Autodesk Inventor part; units mm, degrees
(part 2 of 4)
  line L221 (-47.1334, -28.1027) -> (-48.7956, -28.1027)
  spline S277 degree 2 poles (-48.7956, -28.1027) (-48.7956, -28.5202) (-48.3755, -28.9637) (-48.0021, -28.9637) knots 0 0 0 1 2 2 2
  spline S278 degree 2 poles (-48.0021, -28.9637) (-47.8699, -28.9637) (-47.6131, -28.904) (-47.5094, -28.8574) knots 0 0 0 1 2 2 2
  spline S279 degree 2 poles (-47.5094, -28.8574) (-47.4005, -28.8055) (-47.2501, -28.7147) (-47.2008, -28.6732) knots 0 0 0 1 2 2 2
  line L222 (-47.2008, -28.6732) -> (-47.1775, -28.6732)
  line L223 (-47.1775, -28.6732) -> (-47.1775, -29.1141)
  spline S280 degree 2 poles (-47.1775, -29.1141) (-47.2475, -29.1426) (-47.4601, -29.2256) (-47.5431, -29.2489) knots 0 0 0 1 2 2 2
  spline S281 degree 2 poles (-47.5431, -29.2489) (-47.6598, -29.2826) (-47.8517, -29.3164) (-47.9969, -29.3164) knots 0 0 0 1 2 2 2
  spline S282 degree 2 poles (-47.5276, -27.7941) (-47.5327, -27.6308) (-47.6002, -27.3922) (-47.665, -27.3118) knots 0 0 0 1 2 2 2
  spline S283 degree 2 poles (-47.665, -27.3118) (-47.735, -27.2211) (-47.9554, -27.1251) (-48.1188, -27.1251) knots 0 0 0 1 2 2 2
  spline S284 degree 2 poles (-48.1188, -27.1251) (-48.2796, -27.1251) (-48.5052, -27.2211) (-48.5985, -27.3144) knots 0 0 0 1 2 2 2
  spline S285 degree 2 poles (-48.5985, -27.3144) (-48.6893, -27.4104) (-48.7827, -27.6412) (-48.7956, -27.7941) knots 0 0 0 1 2 2 2
  line L224 (-48.7956, -27.7941) -> (-47.5276, -27.7941)
  line L225 (-45.4504, -27.2937) -> (-45.4712, -27.2937)
  spline S286 degree 2 poles (-45.4712, -27.2937) (-45.5178, -27.2807) (-45.619, -27.2755) (-45.689, -27.2755) knots 0 0 0 1 2 2 2
  spline S287 degree 2 poles (-45.689, -27.2755) (-45.8524, -27.2755) (-46.1739, -27.4181) (-46.3191, -27.5582) knots 0 0 0 1 2 2 2
  line L226 (-46.3191, -27.5582) -> (-46.3191, -29.2619)
  line L227 (-46.3191, -29.2619) -> (-46.7237, -29.2619)
  line L228 (-46.7237, -29.2619) -> (-46.7237, -26.8606)
  line L229 (-46.7237, -26.8606) -> (-46.3191, -26.8606)
  line L230 (-46.3191, -26.8606) -> (-46.3191, -27.2185)
  spline S288 degree 2 poles (-46.3191, -27.2185) (-46.0987, -27.0214) (-45.7694, -26.8606) (-45.6138, -26.8606) knots 0 0 0 1 2 2 2
  spline S289 degree 2 poles (-45.6138, -26.8606) (-45.5515, -26.8606) (-45.4893, -26.8658) (-45.4504, -26.8736) knots 0 0 0 1 2 2 2
  line L231 (-45.4504, -26.8736) -> (-45.4504, -27.2937)
  spline S290 degree 2 poles (-44.4105, -29.3086) (-44.7399, -29.3086) (-45.1107, -28.9326) (-45.1107, -28.5254) knots 0 0 0 1 2 2 2
  line L232 (-45.1107, -28.5254) -> (-45.1107, -27.1951)
  line L233 (-45.1107, -27.1951) -> (-45.383, -27.1951)
  line L234 (-45.383, -27.1951) -> (-45.383, -26.8606)
  line L235 (-45.383, -26.8606) -> (-45.1107, -26.8606)
  line L236 (-45.1107, -26.8606) -> (-45.1107, -26.1708)
  line L237 (-45.1107, -26.1708) -> (-44.7062, -26.1708)
  line L238 (-44.7062, -26.1708) -> (-44.7062, -26.8606)
  line L239 (-44.7062, -26.8606) -> (-43.9619, -26.8606)
  line L240 (-43.9619, -26.8606) -> (-43.9619, -27.1951)
  line L241 (-43.9619, -27.1951) -> (-44.7062, -27.1951)
  line L242 (-44.7062, -27.1951) -> (-44.7062, -28.3387)
  spline S291 degree 2 poles (-44.7062, -28.3387) (-44.7062, -28.5202) (-44.6932, -28.7199) (-44.6491, -28.8055) knots 0 0 0 1 2 2 2
  spline S292 degree 2 poles (-44.6491, -28.8055) (-44.6128, -28.8807) (-44.4494, -28.9559) (-44.3094, -28.9559) knots 0 0 0 1 2 2 2
  spline S293 degree 2 poles (-44.3094, -28.9559) (-44.2109, -28.9559) (-44.0267, -28.8963) (-43.9853, -28.8781) knots 0 0 0 1 2 2 2
  line L243 (-43.9853, -28.8781) -> (-43.9619, -28.8781)
  line L244 (-43.9619, -28.8781) -> (-43.9619, -29.2412)
  spline S294 degree 2 poles (-43.9619, -29.2412) (-44.076, -29.2723) (-44.3094, -29.3086) (-44.4105, -29.3086) knots 0 0 0 1 2 2 2
  spline S295 degree 2 poles (-70.97, -33.6982) (-70.97, -34.1183) (-71.4835, -34.5747) (-71.9165, -34.5747) knots 0 0 0 1 2 2 2
  spline S296 degree 2 poles (-71.9165, -34.5747) (-72.0203, -34.5747) (-72.3652, -34.5384) (-72.4818, -34.5125) knots 0 0 0 1 2 2 2
  line L245 (-72.4818, -34.5125) -> (-72.4818, -34.1027)
  line L246 (-72.4818, -34.1027) -> (-72.4585, -34.1027)
  spline S297 degree 2 poles (-72.4585, -34.1027) (-72.3703, -34.1339) (-72.1084, -34.2065) (-71.9736, -34.2065) knots 0 0 0 1 2 2 2
  spline S298 degree 2 poles (-71.9736, -34.2065) (-71.7765, -34.2065) (-71.5405, -34.1157) (-71.4861, -34.0327) knots 0 0 0 1 2 2 2
  spline S299 degree 2 poles (-71.4861, -34.0327) (-71.4264, -33.9471) (-71.3953, -33.6982) (-71.3953, -33.5348) knots 0 0 0 1 2 2 2
  line L247 (-71.3953, -33.5348) -> (-71.3953, -31.6703)
  line L248 (-71.3953, -31.6703) -> (-72.0721, -31.6703)
  line L249 (-72.0721, -31.6703) -> (-72.0721, -31.3306)
  line L250 (-72.0721, -31.3306) -> (-70.97, -31.3306)
  line L251 (-70.97, -31.3306) -> (-70.97, -33.6982)
  spline S300 degree 2 poles (-68.4002, -33.33) (-68.4002, -33.9368) (-68.9836, -34.598) (-69.4712, -34.598) knots 0 0 0 1 2 2 2
  spline S301 degree 2 poles (-69.4712, -34.598) (-69.9716, -34.598) (-70.5447, -33.916) (-70.5447, -33.33) knots 0 0 0 1 2 2 2
  spline S302 degree 2 poles (-70.5447, -33.33) (-70.5447, -32.7283) (-69.9535, -32.0619) (-69.4712, -32.0619) knots 0 0 0 1 2 2 2
  spline S303 degree 2 poles (-69.4712, -32.0619) (-68.9836, -32.0619) (-68.4002, -32.7257) (-68.4002, -33.33) knots 0 0 0 1 2 2 2
  spline S304 degree 2 poles (-68.8177, -33.33) (-68.8177, -32.8632) (-69.1574, -32.4094) (-69.4712, -32.4094) knots 0 0 0 1 2 2 2
  spline S305 degree 2 poles (-69.4712, -32.4094) (-69.7849, -32.4094) (-70.1272, -32.8632) (-70.1272, -33.33) knots 0 0 0 1 2 2 2
  spline S306 degree 2 poles (-70.1272, -33.33) (-70.1272, -33.7838) (-69.7849, -34.2505) (-69.4712, -34.2505) knots 0 0 0 1 2 2 2
  spline S307 degree 2 poles (-69.4712, -34.2505) (-69.16, -34.2505) (-68.8177, -33.7916) (-68.8177, -33.33) knots 0 0 0 1 2 2 2
  spline S308 degree 2 poles (-66.9428, -34.5851) (-67.5185, -34.5851) (-68.1512, -33.9394) (-68.1512, -33.3429) knots 0 0 0 1 2 2 2
  spline S309 degree 2 poles (-68.1512, -33.3429) (-68.1512, -32.7569) (-67.5366, -32.0619) (-67.0413, -32.0619) knots 0 0 0 1 2 2 2
  spline S310 degree 2 poles (-67.0413, -32.0619) (-66.8183, -32.0619) (-66.4734, -32.1916) (-66.3464, -32.329) knots 0 0 0 1 2 2 2
  spline S311 degree 2 poles (-66.3464, -32.329) (-66.2167, -32.4664) (-66.0793, -32.8632) (-66.0793, -33.151) knots 0 0 0 1 2 2 2
  line L252 (-66.0793, -33.151) -> (-66.0793, -33.3715)
  line L253 (-66.0793, -33.3715) -> (-67.7415, -33.3715)
  spline S312 degree 2 poles (-67.7415, -33.3715) (-67.7415, -33.789) (-67.3214, -34.2324) (-66.948, -34.2324) knots 0 0 0 1 2 2 2
  spline S313 degree 2 poles (-66.948, -34.2324) (-66.8157, -34.2324) (-66.559, -34.1728) (-66.4553, -34.1261) knots 0 0 0 1 2 2 2
  spline S314 degree 2 poles (-66.4553, -34.1261) (-66.3464, -34.0742) (-66.1959, -33.9834) (-66.1467, -33.942) knots 0 0 0 1 2 2 2
  line L254 (-66.1467, -33.942) -> (-66.1233, -33.942)
  line L255 (-66.1233, -33.942) -> (-66.1233, -34.3828)
  spline S315 degree 2 poles (-66.1233, -34.3828) (-66.1934, -34.4113) (-66.406, -34.4943) (-66.489, -34.5176) knots 0 0 0 1 2 2 2
  spline S316 degree 2 poles (-66.489, -34.5176) (-66.6057, -34.5514) (-66.7976, -34.5851) (-66.9428, -34.5851) knots 0 0 0 1 2 2 2
  spline S317 degree 2 poles (-66.4734, -33.0629) (-66.4786, -32.8995) (-66.546, -32.6609) (-66.6109, -32.5805) knots 0 0 0 1 2 2 2
  spline S318 degree 2 poles (-66.6109, -32.5805) (-66.6809, -32.4898) (-66.9013, -32.3938) (-67.0647, -32.3938) knots 0 0 0 1 2 2 2
  spline S319 degree 2 poles (-67.0647, -32.3938) (-67.2254, -32.3938) (-67.4511, -32.4898) (-67.5444, -32.5831) knots 0 0 0 1 2 2 2
  spline S320 degree 2 poles (-67.5444, -32.5831) (-67.6352, -32.6791) (-67.7285, -32.9099) (-67.7415, -33.0629) knots 0 0 0 1 2 2 2
  line L256 (-67.7415, -33.0629) -> (-66.4734, -33.0629)
  line L257 (-65.2572, -34.5306) -> (-65.6618, -34.5306)
  line L258 (-65.6618, -34.5306) -> (-65.6618, -31.188)
  line L259 (-65.6618, -31.188) -> (-65.2572, -31.188)
  line L260 (-65.2572, -31.188) -> (-65.2572, -34.5306)
  spline S321 degree 2 poles (-61.2352, -32.2953) (-61.2352, -32.5027) (-61.383, -32.8762) (-61.5152, -33.0058) knots 0 0 0 1 2 2 2
  spline S322 degree 2 poles (-61.5152, -33.0058) (-61.6812, -33.1692) (-62.1298, -33.3377) (-62.4721, -33.3377) knots 0 0 0 1 2 2 2
  line L261 (-62.4721, -33.3377) -> (-62.8326, -33.3377)
  line L262 (-62.8326, -33.3377) -> (-62.8326, -34.5306)
  line L263 (-62.8326, -34.5306) -> (-63.2579, -34.5306)
  line L264 (-63.2579, -34.5306) -> (-63.2579, -31.3306)
  line L265 (-63.2579, -31.3306) -> (-62.454, -31.3306)
  spline S323 degree 2 poles (-62.454, -31.3306) (-62.1687, -31.3306) (-61.7694, -31.424) (-61.6164, -31.5303) knots 0 0 0 1 2 2 2
  spline S324 degree 2 poles (-61.6164, -31.5303) (-61.4374, -31.6522) (-61.2352, -32.0282) (-61.2352, -32.2953) knots 0 0 0 1 2 2 2
  spline S325 degree 2 poles (-61.6786, -32.3082) (-61.6786, -32.1423) (-61.7927, -31.8985) (-61.9094, -31.8207) knots 0 0 0 1 2 2 2
  spline S326 degree 2 poles (-61.9094, -31.8207) (-62.0105, -31.7533) (-62.2802, -31.6988) (-62.4799, -31.6988) knots 0 0 0 1 2 2 2
  line L266 (-62.4799, -31.6988) -> (-62.8326, -31.6988)
  line L267 (-62.8326, -31.6988) -> (-62.8326, -32.9747)
  line L268 (-62.8326, -32.9747) -> (-62.5421, -32.9747)
  spline S327 degree 2 poles (-62.5421, -32.9747) (-62.2828, -32.9747) (-61.9639, -32.8917) (-61.8601, -32.7828) knots 0 0 0 1 2 2 2
  spline S328 degree 2 poles (-61.8601, -32.7828) (-61.7642, -32.6869) (-61.6786, -32.4612) (-61.6786, -32.3082) knots 0 0 0 1 2 2 2
  line L269 (-60.4494, -34.5306) -> (-60.854, -34.5306)
  line L270 (-60.854, -34.5306) -> (-60.854, -32.1293)
  line L271 (-60.854, -32.1293) -> (-60.4494, -32.1293)
  line L272 (-60.4494, -32.1293) -> (-60.4494, -34.5306)
  line L273 (-60.4209, -31.73) -> (-60.8799, -31.73)
  line L274 (-60.8799, -31.73) -> (-60.8799, -31.3099)
  line L275 (-60.8799, -31.3099) -> (-60.4209, -31.3099)
  line L276 (-60.4209, -31.3099) -> (-60.4209, -31.73)
  spline S329 degree 2 poles (-59.1295, -34.5773) (-59.4588, -34.5773) (-59.8297, -34.2013) (-59.8297, -33.7941) knots 0 0 0 1 2 2 2
  line L277 (-59.8297, -33.7941) -> (-59.8297, -32.4638)
  line L278 (-59.8297, -32.4638) -> (-60.1019, -32.4638)
  line L279 (-60.1019, -32.4638) -> (-60.1019, -32.1293)
  line L280 (-60.1019, -32.1293) -> (-59.8297, -32.1293)
  line L281 (-59.8297, -32.1293) -> (-59.8297, -31.4395)
  line L282 (-59.8297, -31.4395) -> (-59.4251, -31.4395)
  line L283 (-59.4251, -31.4395) -> (-59.4251, -32.1293)
  line L284 (-59.4251, -32.1293) -> (-58.6809, -32.1293)
  line L285 (-58.6809, -32.1293) -> (-58.6809, -32.4638)
  line L286 (-58.6809, -32.4638) -> (-59.4251, -32.4638)
  line L287 (-59.4251, -32.4638) -> (-59.4251, -33.6074)
  spline S330 degree 2 poles (-59.4251, -33.6074) (-59.4251, -33.789) (-59.4122, -33.9886) (-59.3681, -34.0742) knots 0 0 0 1 2 2 2
  spline S331 degree 2 poles (-59.3681, -34.0742) (-59.3318, -34.1494) (-59.1684, -34.2246) (-59.0284, -34.2246) knots 0 0 0 1 2 2 2
  spline S332 degree 2 poles (-59.0284, -34.2246) (-58.9298, -34.2246) (-58.7457, -34.165) (-58.7042, -34.1468) knots 0 0 0 1 2 2 2
  line L288 (-58.7042, -34.1468) -> (-58.6809, -34.1468)
  line L289 (-58.6809, -34.1468) -> (-58.6809, -34.5099)
  spline S333 degree 2 poles (-58.6809, -34.5099) (-58.795, -34.541) (-59.0284, -34.5773) (-59.1295, -34.5773) knots 0 0 0 1 2 2 2
  spline S334 degree 2 poles (-57.0446, -34.2765) (-57.0938, -34.3128) (-57.2598, -34.4424) (-57.3376, -34.4813) knots 0 0 0 1 2 2 2
  spline S335 degree 2 poles (-57.3376, -34.4813) (-57.4439, -34.5384) (-57.6436, -34.598) (-57.8251, -34.598) knots 0 0 0 1 2 2 2
  spline S336 degree 2 poles (-57.8251, -34.598) (-57.9729, -34.598) (-58.24, -34.4865) (-58.3412, -34.3854) knots 0 0 0 1 2 2 2
  spline S337 degree 2 poles (-58.3412, -34.3854) (-58.4371, -34.2869) (-58.5538, -33.9964) (-58.5538, -33.8356) knots 0 0 0 1 2 2 2
  spline S338 degree 2 poles (-58.5538, -33.8356) (-58.5538, -33.5867) (-58.3438, -33.234) (-58.1156, -33.1329) knots 0 0 0 1 2 2 2
  spline S339 degree 2 poles (-58.1156, -33.1329) (-57.9133, -33.0395) (-57.3635, -32.9695) (-57.0446, -32.9514) knots 0 0 0 1 2 2 2
  line L290 (-57.0446, -32.9514) -> (-57.0446, -32.8736)
  spline S340 degree 2 poles (-57.0446, -32.8736) (-57.0446, -32.7335) (-57.1301, -32.5598) (-57.2079, -32.5105) knots 0 0 0 1 2 2 2
  spline S341 degree 2 poles (-57.2079, -32.5105) (-57.2857, -32.4612) (-57.5088, -32.4301) (-57.628, -32.4301) knots 0 0 0 1 2 2 2
  spline S342 degree 2 poles (-57.628, -32.4301) (-57.7681, -32.4301) (-58.1467, -32.5131) (-58.336, -32.5935) knots 0 0 0 1 2 2 2
  line L291 (-58.336, -32.5935) -> (-58.3593, -32.5935)
  line L292 (-58.3593, -32.5935) -> (-58.3593, -32.1812)
  spline S343 degree 2 poles (-58.3593, -32.1812) (-58.2478, -32.1501) (-57.8303, -32.0723) (-57.6254, -32.0723) knots 0 0 0 1 2 2 2
  spline S344 degree 2 poles (-57.6254, -32.0723) (-57.3765, -32.0723) (-57.0368, -32.1501) (-56.9019, -32.2512) knots 0 0 0 1 2 2 2
  spline S345 degree 2 poles (-56.9019, -32.2512) (-56.7697, -32.3497) (-56.64, -32.6635) (-56.64, -32.8891) knots 0 0 0 1 2 2 2
  line L293 (-56.64, -32.8891) -> (-56.64, -34.5306)
  line L294 (-56.64, -34.5306) -> (-57.0446, -34.5306)
  line L295 (-57.0446, -34.5306) -> (-57.0446, -34.2765)
  line L296 (-57.0446, -33.9394) -> (-57.0446, -33.2729)
  spline S346 degree 2 poles (-57.0446, -33.2729) (-57.1898, -33.2859) (-57.628, -33.33) (-57.7655, -33.3715) knots 0 0 0 1 2 2 2
  spline S347 degree 2 poles (-57.7655, -33.3715) (-57.9263, -33.4207) (-58.1363, -33.6256) (-58.1363, -33.8071) knots 0 0 0 1 2 2 2
  spline S348 degree 2 poles (-58.1363, -33.8071) (-58.1363, -34.0146) (-57.9029, -34.2246) (-57.6799, -34.2246) knots 0 0 0 1 2 2 2
  spline S349 degree 2 poles (-57.6799, -34.2246) (-57.4906, -34.2246) (-57.1794, -34.0612) (-57.0446, -33.9394) knots 0 0 0 1 2 2 2
  spline S350 degree 2 poles (-70.97, -38.9669) (-70.97, -39.387) (-71.4835, -39.8434) (-71.9165, -39.8434) knots 0 0 0 1 2 2 2
  spline S351 degree 2 poles (-71.9165, -39.8434) (-72.0203, -39.8434) (-72.3652, -39.8071) (-72.4818, -39.7812) knots 0 0 0 1 2 2 2
  line L297 (-72.4818, -39.7812) -> (-72.4818, -39.3715)
  line L298 (-72.4818, -39.3715) -> (-72.4585, -39.3715)
  spline S352 degree 2 poles (-72.4585, -39.3715) (-72.3703, -39.4026) (-72.1084, -39.4752) (-71.9736, -39.4752) knots 0 0 0 1 2 2 2
  spline S353 degree 2 poles (-71.9736, -39.4752) (-71.7765, -39.4752) (-71.5405, -39.3844) (-71.4861, -39.3014) knots 0 0 0 1 2 2 2
  spline S354 degree 2 poles (-71.4861, -39.3014) (-71.4264, -39.2159) (-71.3953, -38.9669) (-71.3953, -38.8035) knots 0 0 0 1 2 2 2
  line L299 (-71.3953, -38.8035) -> (-71.3953, -36.939)
  line L300 (-71.3953, -36.939) -> (-72.0721, -36.939)
  line L301 (-72.0721, -36.939) -> (-72.0721, -36.5993)
  line L302 (-72.0721, -36.5993) -> (-70.97, -36.5993)
  line L303 (-70.97, -36.5993) -> (-70.97, -38.9669)
  spline S355 degree 2 poles (-68.4002, -38.5987) (-68.4002, -39.2055) (-68.9836, -39.8668) (-69.4712, -39.8668) knots 0 0 0 1 2 2 2
  spline S356 degree 2 poles (-69.4712, -39.8668) (-69.9716, -39.8668) (-70.5447, -39.1847) (-70.5447, -38.5987) knots 0 0 0 1 2 2 2
  spline S357 degree 2 poles (-70.5447, -38.5987) (-70.5447, -37.9971) (-69.9535, -37.3306) (-69.4712, -37.3306) knots 0 0 0 1 2 2 2
  spline S358 degree 2 poles (-69.4712, -37.3306) (-68.9836, -37.3306) (-68.4002, -37.9945) (-68.4002, -38.5987) knots 0 0 0 1 2 2 2
  spline S359 degree 2 poles (-68.8177, -38.5987) (-68.8177, -38.1319) (-69.1574, -37.6781) (-69.4712, -37.6781) knots 0 0 0 1 2 2 2
  spline S360 degree 2 poles (-69.4712, -37.6781) (-69.7849, -37.6781) (-70.1272, -38.1319) (-70.1272, -38.5987) knots 0 0 0 1 2 2 2
  spline S361 degree 2 poles (-70.1272, -38.5987) (-70.1272, -39.0525) (-69.7849, -39.5193) (-69.4712, -39.5193) knots 0 0 0 1 2 2 2
  spline S362 degree 2 poles (-69.4712, -39.5193) (-69.16, -39.5193) (-68.8177, -39.0603) (-68.8177, -38.5987) knots 0 0 0 1 2 2 2
  spline S363 degree 2 poles (-67.337, -39.8564) (-67.5781, -39.8564) (-67.9956, -39.7267) (-68.1331, -39.6541) knots 0 0 0 1 2 2 2
  line L304 (-68.1331, -39.6541) -> (-68.1331, -39.2003)
  line L305 (-68.1331, -39.2003) -> (-68.1123, -39.2003)
  spline S364 degree 2 poles (-68.1123, -39.2003) (-68.0605, -39.2418) (-67.9204, -39.3403) (-67.8037, -39.3948) knots 0 0 0 1 2 2 2
  spline S365 degree 2 poles (-67.8037, -39.3948) (-67.7026, -39.4441) (-67.4536, -39.5167) (-67.3214, -39.5167) knots 0 0 0 1 2 2 2
  spline S366 degree 2 poles (-67.3214, -39.5167) (-67.2254, -39.5167) (-67.005, -39.4726) (-66.9532, -39.4363) knots 0 0 0 1 2 2 2
  spline S367 degree 2 poles (-66.9532, -39.4363) (-66.878, -39.387) (-66.8105, -39.2755) (-66.8105, -39.1614) knots 0 0 0 1 2 2 2
  spline S368 degree 2 poles (-66.8105, -39.1614) (-66.8105, -39.0188) (-66.9661, -38.871) (-67.1658, -38.8217) knots 0 0 0 1 2 2 2
  spline S369 degree 2 poles (-67.1658, -38.8217) (-67.2436, -38.8035) (-67.4925, -38.7517) (-67.5989, -38.7232) knots 0 0 0 1 2 2 2
  spline S370 degree 2 poles (-67.5989, -38.7232) (-67.8737, -38.6428) (-68.1227, -38.3108) (-68.1227, -38.0749) knots 0 0 0 1 2 2 2
  spline S371 degree 2 poles (-68.1227, -38.0749) (-68.1227, -37.7481) (-67.6326, -37.341) (-67.228, -37.341) knots 0 0 0 1 2 2 2
  spline S372 degree 2 poles (-67.228, -37.341) (-67.0284, -37.341) (-66.6238, -37.4395) (-66.4864, -37.5147) knots 0 0 0 1 2 2 2
  line L306 (-66.4864, -37.5147) -> (-66.4864, -37.9478)
  line L307 (-66.4864, -37.9478) -> (-66.5071, -37.9478)
  spline S373 degree 2 poles (-66.5071, -37.9478) (-66.6627, -37.8233) (-67.0413, -37.6807) (-67.2358, -37.6807) knots 0 0 0 1 2 2 2
  spline S374 degree 2 poles (-67.2358, -37.6807) (-67.4355, -37.6807) (-67.7104, -37.8492) (-67.7104, -38.0178) knots 0 0 0 1 2 2 2
  spline S375 degree 2 poles (-67.7104, -38.0178) (-67.7104, -38.1708) (-67.547, -38.3186) (-67.3655, -38.3653) knots 0 0 0 1 2 2 2
  spline S376 degree 2 poles (-67.3655, -38.3653) (-67.2773, -38.3886) (-67.0543, -38.4353) (-66.9324, -38.4638) knots 0 0 0 1 2 2 2
  spline S377 degree 2 poles (-66.9324, -38.4638) (-66.6679, -38.5313) (-66.3982, -38.8398) (-66.3982, -39.1069) knots 0 0 0 1 2 2 2
  spline S378 degree 2 poles (-66.3982, -39.1069) (-66.3982, -39.2625) (-66.5201, -39.5374) (-66.6394, -39.6385) knots 0 0 0 1 2 2 2
  spline S379 degree 2 poles (-66.6394, -39.6385) (-66.7665, -39.7449) (-67.0906, -39.8564) (-67.337, -39.8564) knots 0 0 0 1 2 2 2
  line L308 (-64.137, -39.7993) -> (-64.5415, -39.7993)
  line L309 (-64.5415, -39.7993) -> (-64.5415, -38.4301)
  spline S380 degree 2 poles (-64.5415, -38.4301) (-64.5415, -38.2642) (-64.5726, -37.9789) (-64.6193, -37.8933) knots 0 0 0 1 2 2 2
  spline S381 degree 2 poles (-64.6193, -37.8933) (-64.6686, -37.8026) (-64.8449, -37.7144) (-64.9953, -37.7144) knots 0 0 0 1 2 2 2
  spline S382 degree 2 poles (-64.9953, -37.7144) (-65.1457, -37.7144) (-65.4647, -37.8752) (-65.6177, -38.0048) knots 0 0 0 1 2 2 2
  line L310 (-65.6177, -38.0048) -> (-65.6177, -39.7993)
  line L311 (-65.6177, -39.7993) -> (-66.0222, -39.7993)
  line L312 (-66.0222, -39.7993) -> (-66.0222, -36.4567)
  line L313 (-66.0222, -36.4567) -> (-65.6177, -36.4567)
  line L314 (-65.6177, -36.4567) -> (-65.6177, -37.6651)
  spline S383 degree 2 poles (-65.6177, -37.6651) (-65.4361, -37.5018) (-65.0861, -37.3306) (-64.889, -37.3306) knots 0 0 0 1 2 2 2
  spline S384 degree 2 poles (-64.889, -37.3306) (-64.5363, -37.3306) (-64.137, -37.7974) (-64.137, -38.2408) knots 0 0 0 1 2 2 2
  line L315 (-64.137, -38.2408) -> (-64.137, -39.7993)
  line L316 (-61.7019, -39.7993) -> (-62.1065, -39.7993)
  line L317 (-62.1065, -39.7993) -> (-62.1065, -39.5348)
  spline S385 degree 2 poles (-62.1065, -39.5348) (-62.2932, -39.6982) (-62.6277, -39.8668) (-62.8352, -39.8668) knots 0 0 0 1 2 2 2
  spline S386 degree 2 poles (-62.8352, -39.8668) (-62.9908, -39.8668) (-63.2682, -39.763) (-63.3694, -39.6515) knots 0 0 0 1 2 2 2
  spline S387 degree 2 poles (-63.3694, -39.6515) (-63.4731, -39.54) (-63.5872, -39.2003) (-63.5872, -38.9565) knots 0 0 0 1 2 2 2
  line L318 (-63.5872, -38.9565) -> (-63.5872, -37.398)
  line L319 (-63.5872, -37.398) -> (-63.1827, -37.398)
  line L320 (-63.1827, -37.398) -> (-63.1827, -38.7672)
  spline S388 degree 2 poles (-63.1827, -38.7672) (-63.1827, -38.9591) (-63.1541, -39.2107) (-63.1049, -39.304) knots 0 0 0 1 2 2 2
  spline S389 degree 2 poles (-63.1049, -39.304) (-63.0556, -39.3974) (-62.887, -39.483) (-62.7288, -39.483) knots 0 0 0 1 2 2 2
  spline S390 degree 2 poles (-62.7288, -39.483) (-62.581, -39.483) (-62.2465, -39.3144) (-62.1065, -39.1925) knots 0 0 0 1 2 2 2
  line L321 (-62.1065, -39.1925) -> (-62.1065, -37.398)
  line L322 (-62.1065, -37.398) -> (-61.7019, -37.398)
  line L323 (-61.7019, -37.398) -> (-61.7019, -39.7993)
  spline S391 degree 2 poles (-59.7778, -39.5452) (-59.8271, -39.5815) (-59.993, -39.7112) (-60.0708, -39.7501) knots 0 0 0 1 2 2 2
  spline S392 degree 2 poles (-60.0708, -39.7501) (-60.1771, -39.8071) (-60.3768, -39.8668) (-60.5583, -39.8668) knots 0 0 0 1 2 2 2
  spline S393 degree 2 poles (-60.5583, -39.8668) (-60.7062, -39.8668) (-60.9733, -39.7552) (-61.0744, -39.6541) knots 0 0 0 1 2 2 2
  spline S394 degree 2 poles (-61.0744, -39.6541) (-61.1703, -39.5556) (-61.287, -39.2651) (-61.287, -39.1044) knots 0 0 0 1 2 2 2
  spline S395 degree 2 poles (-61.287, -39.1044) (-61.287, -38.8554) (-61.077, -38.5027) (-60.8488, -38.4016) knots 0 0 0 1 2 2 2
  spline S396 degree 2 poles (-60.8488, -38.4016) (-60.6465, -38.3082) (-60.0968, -38.2382) (-59.7778, -38.2201) knots 0 0 0 1 2 2 2
  line L324 (-59.7778, -38.2201) -> (-59.7778, -38.1423)
  spline S397 degree 2 poles (-59.7778, -38.1423) (-59.7778, -38.0022) (-59.8634, -37.8285) (-59.9412, -37.7792) knots 0 0 0 1 2 2 2
  spline S398 degree 2 poles (-59.9412, -37.7792) (-60.019, -37.73) (-60.242, -37.6988) (-60.3613, -37.6988) knots 0 0 0 1 2 2 2
  spline S399 degree 2 poles (-60.3613, -37.6988) (-60.5013, -37.6988) (-60.8799, -37.7818) (-61.0692, -37.8622) knots 0 0 0 1 2 2 2
  line L325 (-61.0692, -37.8622) -> (-61.0925, -37.8622)
  line L326 (-61.0925, -37.8622) -> (-61.0925, -37.4499)
  spline S400 degree 2 poles (-61.0925, -37.4499) (-60.981, -37.4188) (-60.5635, -37.341) (-60.3587, -37.341) knots 0 0 0 1 2 2 2
  spline S401 degree 2 poles (-60.3587, -37.341) (-60.1097, -37.341) (-59.77, -37.4188) (-59.6352, -37.5199) knots 0 0 0 1 2 2 2
  spline S402 degree 2 poles (-59.6352, -37.5199) (-59.5029, -37.6185) (-59.3733, -37.9322) (-59.3733, -38.1578) knots 0 0 0 1 2 2 2
  line L327 (-59.3733, -38.1578) -> (-59.3733, -39.7993)
  line L328 (-59.3733, -39.7993) -> (-59.7778, -39.7993)
  line L329 (-59.7778, -39.7993) -> (-59.7778, -39.5452)
  line L330 (-59.7778, -39.2081) -> (-59.7778, -38.5416)
  spline S403 degree 2 poles (-59.7778, -38.5416) (-59.923, -38.5546) (-60.3613, -38.5987) (-60.4987, -38.6402) knots 0 0 0 1 2 2 2
  spline S404 degree 2 poles (-60.4987, -38.6402) (-60.6595, -38.6894) (-60.8695, -38.8943) (-60.8695, -39.0758) knots 0 0 0 1 2 2 2
  spline S405 degree 2 poles (-60.8695, -39.0758) (-60.8695, -39.2833) (-60.6361, -39.4933) (-60.4131, -39.4933) knots 0 0 0 1 2 2 2
  spline S406 degree 2 poles (-60.4131, -39.4933) (-60.2238, -39.4933) (-59.9126, -39.33) (-59.7778, -39.2081) knots 0 0 0 1 2 2 2
  line L331 (-55.066, -39.7993) -> (-55.6183, -39.7993)
  line L332 (-55.6183, -39.7993) -> (-56.7878, -38.3108)
  line L333 (-56.7878, -38.3108) -> (-56.9746, -38.5209)
  line L334 (-56.9746, -38.5209) -> (-56.9746, -39.7993)
  line L335 (-56.9746, -39.7993) -> (-57.3998, -39.7993)
  line L336 (-57.3998, -39.7993) -> (-57.3998, -36.5993)
  line L337 (-57.3998, -36.5993) -> (-56.9746, -36.5993)
  line L338 (-56.9746, -36.5993) -> (-56.9746, -38.0697)
  line L339 (-56.9746, -38.0697) -> (-55.6624, -36.5993)
  line L340 (-55.6624, -36.5993) -> (-55.1438, -36.5993)
  line L341 (-55.1438, -36.5993) -> (-56.4689, -38.0282)
  line L342 (-56.4689, -38.0282) -> (-55.066, -39.7993)
  spline S407 degree 2 poles (-53.5049, -39.5452) (-53.5541, -39.5815) (-53.7201, -39.7112) (-53.7979, -39.7501) knots 0 0 0 1 2 2 2
  spline S408 degree 2 poles (-53.7979, -39.7501) (-53.9042, -39.8071) (-54.1039, -39.8668) (-54.2854, -39.8668) knots 0 0 0 1 2 2 2
  spline S409 degree 2 poles (-54.2854, -39.8668) (-54.4332, -39.8668) (-54.7003, -39.7552) (-54.8015, -39.6541) knots 0 0 0 1 2 2 2
  spline S410 degree 2 poles (-54.8015, -39.6541) (-54.8974, -39.5556) (-55.0141, -39.2651) (-55.0141, -39.1044) knots 0 0 0 1 2 2 2
  spline S411 degree 2 poles (-55.0141, -39.1044) (-55.0141, -38.8554) (-54.8041, -38.5027) (-54.5759, -38.4016) knots 0 0 0 1 2 2 2
  spline S412 degree 2 poles (-54.5759, -38.4016) (-54.3736, -38.3082) (-53.8238, -38.2382) (-53.5049, -38.2201) knots 0 0 0 1 2 2 2
  line L343 (-53.5049, -38.2201) -> (-53.5049, -38.1423)
  spline S413 degree 2 poles (-53.5049, -38.1423) (-53.5049, -38.0022) (-53.5904, -37.8285) (-53.6682, -37.7792) knots 0 0 0 1 2 2 2
  spline S414 degree 2 poles (-53.6682, -37.7792) (-53.746, -37.73) (-53.969, -37.6988) (-54.0883, -37.6988) knots 0 0 0 1 2 2 2
  spline S415 degree 2 poles (-54.0883, -37.6988) (-54.2284, -37.6988) (-54.607, -37.7818) (-54.7963, -37.8622) knots 0 0 0 1 2 2 2
  line L344 (-54.7963, -37.8622) -> (-54.8196, -37.8622)
  line L345 (-54.8196, -37.8622) -> (-54.8196, -37.4499)
  spline S416 degree 2 poles (-54.8196, -37.4499) (-54.7081, -37.4188) (-54.2906, -37.341) (-54.0857, -37.341) knots 0 0 0 1 2 2 2
  spline S417 degree 2 poles (-54.0857, -37.341) (-53.8368, -37.341) (-53.4971, -37.4188) (-53.3622, -37.5199) knots 0 0 0 1 2 2 2
  spline S418 degree 2 poles (-53.3622, -37.5199) (-53.23, -37.6185) (-53.1003, -37.9322) (-53.1003, -38.1578) knots 0 0 0 1 2 2 2
  line L346 (-53.1003, -38.1578) -> (-53.1003, -39.7993)
  line L347 (-53.1003, -39.7993) -> (-53.5049, -39.7993)
  line L348 (-53.5049, -39.7993) -> (-53.5049, -39.5452)
  line L349 (-53.5049, -39.2081) -> (-53.5049, -38.5416)
  spline S419 degree 2 poles (-53.5049, -38.5416) (-53.6501, -38.5546) (-54.0883, -38.5987) (-54.2258, -38.6402) knots 0 0 0 1 2 2 2
  spline S420 degree 2 poles (-54.2258, -38.6402) (-54.3865, -38.6894) (-54.5966, -38.8943) (-54.5966, -39.0758) knots 0 0 0 1 2 2 2
  spline S421 degree 2 poles (-54.5966, -39.0758) (-54.5966, -39.2833) (-54.3632, -39.4933) (-54.1402, -39.4933) knots 0 0 0 1 2 2 2
  spline S422 degree 2 poles (-54.1402, -39.4933) (-53.9509, -39.4933) (-53.6397, -39.33) (-53.5049, -39.2081) knots 0 0 0 1 2 2 2
  spline S423 degree 2 poles (-50.5201, -38.5338) (-50.5201, -39.1355) (-51.0932, -39.846) (-51.5314, -39.846) knots 0 0 0 1 2 2 2
  spline S424 degree 2 poles (-51.5314, -39.846) (-51.7104, -39.846) (-51.9853, -39.763) (-52.1279, -39.6774) knots 0 0 0 1 2 2 2
  line L350 (-52.1279, -39.6774) -> (-52.1279, -40.6836)
  line L351 (-52.1279, -40.6836) -> (-52.5324, -40.6836)
  line L352 (-52.5324, -40.6836) -> (-52.5324, -37.398)
  line L353 (-52.5324, -37.398) -> (-52.1279, -37.398)
  line L354 (-52.1279, -37.398) -> (-52.1279, -37.6496)
  spline S425 degree 2 poles (-52.1279, -37.6496) (-51.9775, -37.5121) (-51.6092, -37.3306) (-51.394, -37.3306) knots 0 0 0 1 2 2 2
  spline S426 degree 2 poles (-51.394, -37.3306) (-50.9817, -37.3306) (-50.5201, -37.9841) (-50.5201, -38.5338) knots 0 0 0 1 2 2 2
  spline S427 degree 2 poles (-50.9376, -38.5805) (-50.9376, -38.1682) (-51.1995, -37.7144) (-51.4925, -37.7144) knots 0 0 0 1 2 2 2
  spline S428 degree 2 poles (-51.4925, -37.7144) (-51.6637, -37.7144) (-51.9853, -37.8674) (-52.1279, -37.9867) knots 0 0 0 1 2 2 2
  line L355 (-52.1279, -37.9867) -> (-52.1279, -39.3507)
  spline S429 degree 2 poles (-52.1279, -39.3507) (-51.9697, -39.4259) (-51.7441, -39.483) (-51.5989, -39.483) knots 0 0 0 1 2 2 2
  spline S430 degree 2 poles (-51.5989, -39.483) (-51.2851, -39.483) (-50.9376, -39.0214) (-50.9376, -38.5805) knots 0 0 0 1 2 2 2
  line L356 (-48.2329, -39.7993) -> (-48.6374, -39.7993)
  line L357 (-48.6374, -39.7993) -> (-48.6374, -39.5348)
  spline S431 degree 2 poles (-48.6374, -39.5348) (-48.8241, -39.6982) (-49.1587, -39.8668) (-49.3661, -39.8668) knots 0 0 0 1 2 2 2
  spline S432 degree 2 poles (-49.3661, -39.8668) (-49.5217, -39.8668) (-49.7992, -39.763) (-49.9003, -39.6515) knots 0 0 0 1 2 2 2
  spline S433 degree 2 poles (-49.9003, -39.6515) (-50.0041, -39.54) (-50.1182, -39.2003) (-50.1182, -38.9565) knots 0 0 0 1 2 2 2
  line L358 (-50.1182, -38.9565) -> (-50.1182, -37.398)
  line L359 (-50.1182, -37.398) -> (-49.7136, -37.398)
  line L360 (-49.7136, -37.398) -> (-49.7136, -38.7672)
  spline S434 degree 2 poles (-49.7136, -38.7672) (-49.7136, -38.9591) (-49.6851, -39.2107) (-49.6358, -39.304) knots 0 0 0 1 2 2 2
  spline S435 degree 2 poles (-49.6358, -39.304) (-49.5865, -39.3974) (-49.418, -39.483) (-49.2598, -39.483) knots 0 0 0 1 2 2 2
  spline S436 degree 2 poles (-49.2598, -39.483) (-49.112, -39.483) (-48.7775, -39.3144) (-48.6374, -39.1925) knots 0 0 0 1 2 2 2
  line L361 (-48.6374, -39.1925) -> (-48.6374, -37.398)
  line L362 (-48.6374, -37.398) -> (-48.2329, -37.398)
  line L363 (-48.2329, -37.398) -> (-48.2329, -39.7993)
  spline S437 degree 2 poles (-46.9985, -39.8564) (-47.2397, -39.8564) (-47.6572, -39.7267) (-47.7947, -39.6541) knots 0 0 0 1 2 2 2
  line L364 (-47.7947, -39.6541) -> (-47.7947, -39.2003)
  line L365 (-47.7947, -39.2003) -> (-47.7739, -39.2003)
  spline S438 degree 2 poles (-47.7739, -39.2003) (-47.722, -39.2418) (-47.582, -39.3403) (-47.4653, -39.3948) knots 0 0 0 1 2 2 2
  spline S439 degree 2 poles (-47.4653, -39.3948) (-47.3642, -39.4441) (-47.1152, -39.5167) (-46.983, -39.5167) knots 0 0 0 1 2 2 2
  spline S440 degree 2 poles (-46.983, -39.5167) (-46.887, -39.5167) (-46.6666, -39.4726) (-46.6147, -39.4363) knots 0 0 0 1 2 2 2
  spline S441 degree 2 poles (-46.6147, -39.4363) (-46.5395, -39.387) (-46.4721, -39.2755) (-46.4721, -39.1614) knots 0 0 0 1 2 2 2
  spline S442 degree 2 poles (-46.4721, -39.1614) (-46.4721, -39.0188) (-46.6277, -38.871) (-46.8274, -38.8217) knots 0 0 0 1 2 2 2
  spline S443 degree 2 poles (-46.8274, -38.8217) (-46.9052, -38.8035) (-47.1541, -38.7517) (-47.2605, -38.7232) knots 0 0 0 1 2 2 2
  spline S444 degree 2 poles (-47.2605, -38.7232) (-47.5353, -38.6428) (-47.7843, -38.3108) (-47.7843, -38.0749) knots 0 0 0 1 2 2 2
  spline S445 degree 2 poles (-47.7843, -38.0749) (-47.7843, -37.7481) (-47.2942, -37.341) (-46.8896, -37.341) knots 0 0 0 1 2 2 2
  spline S446 degree 2 poles (-46.8896, -37.341) (-46.69, -37.341) (-46.2854, -37.4395) (-46.148, -37.5147) knots 0 0 0 1 2 2 2
  line L366 (-46.148, -37.5147) -> (-46.148, -37.9478)
  line L367 (-46.148, -37.9478) -> (-46.1687, -37.9478)
  spline S447 degree 2 poles (-46.1687, -37.9478) (-46.3243, -37.8233) (-46.7029, -37.6807) (-46.8974, -37.6807) knots 0 0 0 1 2 2 2
  spline S448 degree 2 poles (-46.8974, -37.6807) (-47.0971, -37.6807) (-47.372, -37.8492) (-47.372, -38.0178) knots 0 0 0 1 2 2 2
  spline S449 degree 2 poles (-47.372, -38.0178) (-47.372, -38.1708) (-47.2086, -38.3186) (-47.0271, -38.3653) knots 0 0 0 1 2 2 2
  spline S450 degree 2 poles (-47.0271, -38.3653) (-46.9389, -38.3886) (-46.7159, -38.4353) (-46.594, -38.4638) knots 0 0 0 1 2 2 2
  spline S451 degree 2 poles (-46.594, -38.4638) (-46.3295, -38.5313) (-46.0598, -38.8398) (-46.0598, -39.1069) knots 0 0 0 1 2 2 2
  spline S452 degree 2 poles (-46.0598, -39.1069) (-46.0598, -39.2625) (-46.1817, -39.5374) (-46.301, -39.6385) knots 0 0 0 1 2 2 2
  spline S453 degree 2 poles (-46.301, -39.6385) (-46.428, -39.7449) (-46.7522, -39.8564) (-46.9985, -39.8564) knots 0 0 0 1 2 2 2
  spline S454 degree 2 poles (-44.3457, -39.5452) (-44.395, -39.5815) (-44.5609, -39.7112) (-44.6387, -39.7501) knots 0 0 0 1 2 2 2
  spline S455 degree 2 poles (-44.6387, -39.7501) (-44.7451, -39.8071) (-44.9447, -39.8668) (-45.1263, -39.8668) knots 0 0 0 1 2 2 2
  spline S456 degree 2 poles (-45.1263, -39.8668) (-45.2741, -39.8668) (-45.5412, -39.7552) (-45.6423, -39.6541) knots 0 0 0 1 2 2 2
  spline S457 degree 2 poles (-45.6423, -39.6541) (-45.7383, -39.5556) (-45.8549, -39.2651) (-45.8549, -39.1044) knots 0 0 0 1 2 2 2
  spline S458 degree 2 poles (-45.8549, -39.1044) (-45.8549, -38.8554) (-45.6449, -38.5027) (-45.4167, -38.4016) knots 0 0 0 1 2 2 2
  spline S459 degree 2 poles (-45.4167, -38.4016) (-45.2144, -38.3082) (-44.6647, -38.2382) (-44.3457, -38.2201) knots 0 0 0 1 2 2 2
  line L368 (-44.3457, -38.2201) -> (-44.3457, -38.1423)
  spline S460 degree 2 poles (-44.3457, -38.1423) (-44.3457, -38.0022) (-44.4313, -37.8285) (-44.5091, -37.7792) knots 0 0 0 1 2 2 2
  spline S461 degree 2 poles (-44.5091, -37.7792) (-44.5869, -37.73) (-44.8099, -37.6988) (-44.9292, -37.6988) knots 0 0 0 1 2 2 2
  spline S462 degree 2 poles (-44.9292, -37.6988) (-45.0692, -37.6988) (-45.4478, -37.7818) (-45.6371, -37.8622) knots 0 0 0 1 2 2 2
  line L369 (-45.6371, -37.8622) -> (-45.6605, -37.8622)
  line L370 (-45.6605, -37.8622) -> (-45.6605, -37.4499)
  spline S463 degree 2 poles (-45.6605, -37.4499) (-45.5489, -37.4188) (-45.1314, -37.341) (-44.9266, -37.341) knots 0 0 0 1 2 2 2
  spline S464 degree 2 poles (-44.9266, -37.341) (-44.6776, -37.341) (-44.3379, -37.4188) (-44.2031, -37.5199) knots 0 0 0 1 2 2 2
  spline S465 degree 2 poles (-44.2031, -37.5199) (-44.0708, -37.6185) (-43.9412, -37.9322) (-43.9412, -38.1578) knots 0 0 0 1 2 2 2
  line L371 (-43.9412, -38.1578) -> (-43.9412, -39.7993)
  line L372 (-43.9412, -39.7993) -> (-44.3457, -39.7993)
  line L373 (-44.3457, -39.7993) -> (-44.3457, -39.5452)
  line L374 (-44.3457, -39.2081) -> (-44.3457, -38.5416)
  spline S466 degree 2 poles (-44.3457, -38.5416) (-44.4909, -38.5546) (-44.9292, -38.5987) (-45.0666, -38.6402) knots 0 0 0 1 2 2 2
  spline S467 degree 2 poles (-45.0666, -38.6402) (-45.2274, -38.6894) (-45.4374, -38.8943) (-45.4374, -39.0758) knots 0 0 0 1 2 2 2
  spline S468 degree 2 poles (-45.4374, -39.0758) (-45.4374, -39.2833) (-45.2041, -39.4933) (-44.981, -39.4933) knots 0 0 0 1 2 2 2
  spline S469 degree 2 poles (-44.981, -39.4933) (-44.7917, -39.4933) (-44.4806, -39.33) (-44.3457, -39.2081) knots 0 0 0 1 2 2 2
  line L375 (-41.488, -39.7993) -> (-41.8925, -39.7993)
  line L376 (-41.8925, -39.7993) -> (-41.8925, -38.4301)
  spline S470 degree 2 poles (-41.8925, -38.4301) (-41.8925, -38.2642) (-41.9237, -37.9789) (-41.9703, -37.8933) knots 0 0 0 1 2 2 2
  spline S471 degree 2 poles (-41.9703, -37.8933) (-42.0196, -37.8026) (-42.1959, -37.7144) (-42.3464, -37.7144) knots 0 0 0 1 2 2 2
  spline S472 degree 2 poles (-42.3464, -37.7144) (-42.4968, -37.7144) (-42.8157, -37.8752) (-42.9687, -38.0048) knots 0 0 0 1 2 2 2
  line L377 (-42.9687, -38.0048) -> (-42.9687, -39.7993)
  line L378 (-42.9687, -39.7993) -> (-43.3733, -39.7993)
  line L379 (-43.3733, -39.7993) -> (-43.3733, -37.398)
  line L380 (-43.3733, -37.398) -> (-42.9687, -37.398)
  line L381 (-42.9687, -37.398) -> (-42.9687, -37.6651)
  spline S473 degree 2 poles (-42.9687, -37.6651) (-42.7872, -37.5018) (-42.4371, -37.3306) (-42.24, -37.3306) knots 0 0 0 1 2 2 2
  spline S474 degree 2 poles (-42.24, -37.3306) (-41.8874, -37.3306) (-41.488, -37.7974) (-41.488, -38.2408) knots 0 0 0 1 2 2 2
  line L382 (-41.488, -38.2408) -> (-41.488, -39.7993)
  spline S475 degree 2 poles (-39.582, -39.5452) (-39.6313, -39.5815) (-39.7972, -39.7112) (-39.875, -39.7501) knots 0 0 0 1 2 2 2
  spline S476 degree 2 poles (-39.875, -39.7501) (-39.9814, -39.8071) (-40.181, -39.8668) (-40.3626, -39.8668) knots 0 0 0 1 2 2 2
  spline S477 degree 2 poles (-40.3626, -39.8668) (-40.5104, -39.8668) (-40.7775, -39.7552) (-40.8786, -39.6541) knots 0 0 0 1 2 2 2
  spline S478 degree 2 poles (-40.8786, -39.6541) (-40.9746, -39.5556) (-41.0912, -39.2651) (-41.0912, -39.1044) knots 0 0 0 1 2 2 2
  spline S479 degree 2 poles (-41.0912, -39.1044) (-41.0912, -38.8554) (-40.8812, -38.5027) (-40.653, -38.4016) knots 0 0 0 1 2 2 2
  spline S480 degree 2 poles (-40.653, -38.4016) (-40.4507, -38.3082) (-39.901, -38.2382) (-39.582, -38.2201) knots 0 0 0 1 2 2 2
  line L383 (-39.582, -38.2201) -> (-39.582, -38.1423)
  spline S481 degree 2 poles (-39.582, -38.1423) (-39.582, -38.0022) (-39.6676, -37.8285) (-39.7454, -37.7792) knots 0 0 0 1 2 2 2
  spline S482 degree 2 poles (-39.7454, -37.7792) (-39.8232, -37.73) (-40.0462, -37.6988) (-40.1655, -37.6988) knots 0 0 0 1 2 2 2
  spline S483 degree 2 poles (-40.1655, -37.6988) (-40.3055, -37.6988) (-40.6841, -37.7818) (-40.8734, -37.8622) knots 0 0 0 1 2 2 2
  line L384 (-40.8734, -37.8622) -> (-40.8968, -37.8622)
  line L385 (-40.8968, -37.8622) -> (-40.8968, -37.4499)
  spline S484 degree 2 poles (-40.8968, -37.4499) (-40.7853, -37.4188) (-40.3677, -37.341) (-40.1629, -37.341) knots 0 0 0 1 2 2 2
  spline S485 degree 2 poles (-40.1629, -37.341) (-39.9139, -37.341) (-39.5742, -37.4188) (-39.4394, -37.5199) knots 0 0 0 1 2 2 2
  spline S486 degree 2 poles (-39.4394, -37.5199) (-39.3071, -37.6185) (-39.1775, -37.9322) (-39.1775, -38.1578) knots 0 0 0 1 2 2 2
  line L386 (-39.1775, -38.1578) -> (-39.1775, -39.7993)
  line L387 (-39.1775, -39.7993) -> (-39.582, -39.7993)
  line L388 (-39.582, -39.7993) -> (-39.582, -39.5452)
  line L389 (-39.582, -39.2081) -> (-39.582, -38.5416)
  spline S487 degree 2 poles (-39.582, -38.5416) (-39.7272, -38.5546) (-40.1655, -38.5987) (-40.3029, -38.6402) knots 0 0 0 1 2 2 2
  spline S488 degree 2 poles (-40.3029, -38.6402) (-40.4637, -38.6894) (-40.6737, -38.8943) (-40.6737, -39.0758) knots 0 0 0 1 2 2 2
  spline S489 degree 2 poles (-40.6737, -39.0758) (-40.6737, -39.2833) (-40.4404, -39.4933) (-40.2173, -39.4933) knots 0 0 0 1 2 2 2
  spline S490 degree 2 poles (-40.2173, -39.4933) (-40.028, -39.4933) (-39.7169, -39.33) (-39.582, -39.2081) knots 0 0 0 1 2 2 2
  spline S491 degree 2 poles (-71.2838, -45.1251) (-71.6313, -45.1251) (-72.1188, -44.9799) (-72.334, -44.8761) knots 0 0 0 1 2 2 2
  line L390 (-72.334, -44.8761) -> (-72.334, -44.3419)
  line L391 (-72.334, -44.3419) -> (-72.3029, -44.3419)
  spline S492 degree 2 poles (-72.3029, -44.3419) (-72.0929, -44.539) (-71.5613, -44.7569) (-71.3149, -44.7569) knots 0 0 0 1 2 2 2
  spline S493 degree 2 poles (-71.3149, -44.7569) (-70.9622, -44.7569) (-70.6018, -44.4638) (-70.6018, -44.2227) knots 0 0 0 1 2 2 2
  spline S494 degree 2 poles (-70.6018, -44.2227) (-70.6018, -44.0308) (-70.7911, -43.7922) (-70.9959, -43.7325) knots 0 0 0 1 2 2 2
  spline S495 degree 2 poles (-70.9959, -43.7325) (-71.1438, -43.6911) (-71.3901, -43.634) (-71.5742, -43.5873) knots 0 0 0 1 2 2 2
  spline S496 degree 2 poles (-71.5742, -43.5873) (-71.7402, -43.5432) (-72.0021, -43.411) (-72.1032, -43.3047) knots 0 0 0 1 2 2 2
  spline S497 degree 2 poles (-72.1032, -43.3047) (-72.2018, -43.1984) (-72.3107, -42.9131) (-72.3107, -42.7264) knots 0 0 0 1 2 2 2
  spline S498 degree 2 poles (-72.3107, -42.7264) (-72.3107, -42.3374) (-71.7039, -41.811) (-71.2345, -41.811) knots 0 0 0 1 2 2 2
  spline S499 degree 2 poles (-71.2345, -41.811) (-70.9648, -41.811) (-70.4877, -41.9173) (-70.2828, -42.0184) knots 0 0 0 1 2 2 2
  line L392 (-70.2828, -42.0184) -> (-70.2828, -42.5267)
  line L393 (-70.2828, -42.5267) -> (-70.3139, -42.5267)
  spline S500 degree 2 poles (-70.3139, -42.5267) (-70.4669, -42.3867) (-70.9441, -42.1792) (-71.206, -42.1792) knots 0 0 0 1 2 2 2
  spline S501 degree 2 poles (-71.206, -42.1792) (-71.5016, -42.1792) (-71.8673, -42.4567) (-71.8673, -42.6823) knots 0 0 0 1 2 2 2
  spline S502 degree 2 poles (-71.8673, -42.6823) (-71.8673, -42.8846) (-71.652, -43.1257) (-71.4498, -43.1802) knots 0 0 0 1 2 2 2
  spline S503 degree 2 poles (-71.4498, -43.1802) (-71.3149, -43.2165) (-70.9233, -43.3099) (-70.7937, -43.3488) knots 0 0 0 1 2 2 2
  spline S504 degree 2 poles (-70.7937, -43.3488) (-70.4643, -43.4499) (-70.1583, -43.857) (-70.1583, -44.1552) knots 0 0 0 1 2 2 2
  spline S505 degree 2 poles (-70.1583, -44.1552) (-70.1583, -44.3445) (-70.3113, -44.7076) (-70.4488, -44.8347) knots 0 0 0 1 2 2 2
  spline S506 degree 2 poles (-70.4488, -44.8347) (-70.6018, -44.9747) (-70.9908, -45.1251) (-71.2838, -45.1251) knots 0 0 0 1 2 2 2
  line L394 (-69.3441, -45.068) -> (-69.7486, -45.068)
  line L395 (-69.7486, -45.068) -> (-69.7486, -42.6667)
  line L396 (-69.7486, -42.6667) -> (-69.3441, -42.6667)
  line L397 (-69.3441, -42.6667) -> (-69.3441, -45.068)
  line L398 (-69.3156, -42.2674) -> (-69.7746, -42.2674)
  line L399 (-69.7746, -42.2674) -> (-69.7746, -41.8473)
  line L400 (-69.7746, -41.8473) -> (-69.3156, -41.8473)
  line L401 (-69.3156, -41.8473) -> (-69.3156, -42.2674)
  line L402 (-66.0274, -45.068) -> (-66.0274, -43.6781)
  spline S507 degree 2 poles (-66.0274, -43.6781) (-66.0274, -43.5121) (-66.0533, -43.2295) (-66.0948, -43.1517) knots 0 0 0 1 2 2 2
  spline S508 degree 2 poles (-66.0948, -43.1517) (-66.1363, -43.0661) (-66.2945, -42.9831) (-66.4319, -42.9831) knots 0 0 0 1 2 2 2
  spline S509 degree 2 poles (-66.4319, -42.9831) (-66.5564, -42.9831) (-66.8417, -43.1361) (-66.9921, -43.2813) knots 0 0 0 1 2 2 2
  spline S510 degree 2 poles (-66.9921, -43.2813) (-66.9895, -43.3176) (-66.9843, -43.4188) (-66.9843, -43.4862) knots 0 0 0 1 2 2 2
  line L403 (-66.9843, -43.4862) -> (-66.9843, -45.068)
  line L404 (-66.9843, -45.068) -> (-67.3888, -45.068)
  line L405 (-67.3888, -45.068) -> (-67.3888, -43.6781)
  spline S511 degree 2 poles (-67.3888, -43.6781) (-67.3888, -43.5121) (-67.4147, -43.2295) (-67.4562, -43.1517) knots 0 0 0 1 2 2 2
  spline S512 degree 2 poles (-67.4562, -43.1517) (-67.4977, -43.0661) (-67.6559, -42.9831) (-67.7934, -42.9831) knots 0 0 0 1 2 2 2
  spline S513 degree 2 poles (-67.7934, -42.9831) (-67.923, -42.9831) (-68.2109, -43.1465) (-68.3457, -43.2736) knots 0 0 0 1 2 2 2
  line L406 (-68.3457, -43.2736) -> (-68.3457, -45.068)
  line L407 (-68.3457, -45.068) -> (-68.7502, -45.068)
  line L408 (-68.7502, -45.068) -> (-68.7502, -42.6667)
  line L409 (-68.7502, -42.6667) -> (-68.3457, -42.6667)
  line L410 (-68.3457, -42.6667) -> (-68.3457, -42.9313)
  spline S514 degree 2 poles (-68.3457, -42.9313) (-68.1875, -42.7731) (-67.8763, -42.5993) (-67.6896, -42.5993) knots 0 0 0 1 2 2 2
  spline S515 degree 2 poles (-67.6896, -42.5993) (-67.477, -42.5993) (-67.1477, -42.7938) (-67.0621, -43.0142) knots 0 0 0 1 2 2 2
  spline S516 degree 2 poles (-67.0621, -43.0142) (-66.878, -42.8094) (-66.5305, -42.5993) (-66.3282, -42.5993) knots 0 0 0 1 2 2 2
  spline S517 degree 2 poles (-66.3282, -42.5993) (-66.1726, -42.5993) (-65.9185, -42.6953) (-65.8251, -42.8042) knots 0 0 0 1 2 2 2
  spline S518 degree 2 poles (-65.8251, -42.8042) (-65.7292, -42.9131) (-65.6229, -43.2398) (-65.6229, -43.4862) knots 0 0 0 1 2 2 2
  line L411 (-65.6229, -43.4862) -> (-65.6229, -45.068)
  line L412 (-65.6229, -45.068) -> (-66.0274, -45.068)
  line L413 (-62.1454, -42.6667) -> (-62.7548, -45.068)
  line L414 (-62.7548, -45.068) -> (-63.1282, -45.068)
  line L415 (-63.1282, -45.068) -> (-63.7143, -43.2165)
  line L416 (-63.7143, -43.2165) -> (-64.2977, -45.068)
  line L417 (-64.2977, -45.068) -> (-64.6686, -45.068)
  line L418 (-64.6686, -45.068) -> (-65.2831, -42.6667)
  line L419 (-65.2831, -42.6667) -> (-64.863, -42.6667)
  line L420 (-64.863, -42.6667) -> (-64.4378, -44.5261)
  line L421 (-64.4378, -44.5261) -> (-63.8699, -42.6667)
  line L422 (-63.8699, -42.6667) -> (-63.5353, -42.6667)
  line L423 (-63.5353, -42.6667) -> (-62.9519, -44.5261)
  line L424 (-62.9519, -44.5261) -> (-62.5525, -42.6667)
  line L425 (-62.5525, -42.6667) -> (-62.1454, -42.6667)
  line L426 (-61.3778, -45.068) -> (-61.7823, -45.068)
  line L427 (-61.7823, -45.068) -> (-61.7823, -42.6667)
  line L428 (-61.7823, -42.6667) -> (-61.3778, -42.6667)
  line L429 (-61.3778, -42.6667) -> (-61.3778, -45.068)
  line L430 (-61.3493, -42.2674) -> (-61.8083, -42.2674)
  line L431 (-61.8083, -42.2674) -> (-61.8083, -41.8473)
  line L432 (-61.8083, -41.8473) -> (-61.3493, -41.8473)
  line L433 (-61.3493, -41.8473) -> (-61.3493, -42.2674)
  line L434 (-58.8987, -45.068) -> (-59.3032, -45.068)
  line L435 (-59.3032, -45.068) -> (-59.3032, -43.6988)
  spline S519 degree 2 poles (-59.3032, -43.6988) (-59.3032, -43.5329) (-59.3344, -43.2476) (-59.381, -43.162) knots 0 0 0 1 2 2 2
  spline S520 degree 2 poles (-59.381, -43.162) (-59.4303, -43.0713) (-59.6066, -42.9831) (-59.7571, -42.9831) knots 0 0 0 1 2 2 2
  spline S521 degree 2 poles (-59.7571, -42.9831) (-59.9075, -42.9831) (-60.2264, -43.1439) (-60.3794, -43.2736) knots 0 0 0 1 2 2 2
  line L436 (-60.3794, -43.2736) -> (-60.3794, -45.068)
  line L437 (-60.3794, -45.068) -> (-60.784, -45.068)
  line L438 (-60.784, -45.068) -> (-60.784, -42.6667)
  line L439 (-60.784, -42.6667) -> (-60.3794, -42.6667)
  line L440 (-60.3794, -42.6667) -> (-60.3794, -42.9338)
  spline S522 degree 2 poles (-60.3794, -42.9338) (-60.1979, -42.7705) (-59.8478, -42.5993) (-59.6507, -42.5993) knots 0 0 0 1 2 2 2
  spline S523 degree 2 poles (-59.6507, -42.5993) (-59.2981, -42.5993) (-58.8987, -43.0661) (-58.8987, -43.5095) knots 0 0 0 1 2 2 2
  line L441 (-58.8987, -43.5095) -> (-58.8987, -45.068)
  spline S524 degree 2 poles (-57.6773, -45.1355) (-57.6773, -45.5452) (-58.1182, -45.9757) (-58.5045, -45.9757) knots 0 0 0 1 2 2 2
  spline S525 degree 2 poles (-58.5045, -45.9757) (-58.572, -45.9757) (-58.7379, -45.9627) (-58.8183, -45.9497) knots 0 0 0 1 2 2 2
  line L442 (-58.8183, -45.9497) -> (-58.8183, -45.5867)
  line L443 (-58.8183, -45.5867) -> (-58.795, -45.5867)
  spline S526 degree 2 poles (-58.795, -45.5867) (-58.7483, -45.5971) (-58.6342, -45.6178) (-58.5823, -45.6178) knots 0 0 0 1 2 2 2
  spline S527 degree 2 poles (-58.5823, -45.6178) (-58.4216, -45.6178) (-58.2115, -45.5374) (-58.1622, -45.4518) knots 0 0 0 1 2 2 2
  spline S528 degree 2 poles (-58.1622, -45.4518) (-58.113, -45.374) (-58.0818, -45.1381) (-58.0818, -44.9695) knots 0 0 0 1 2 2 2
  line L444 (-58.0818, -44.9695) -> (-58.0818, -43.0013)
  line L445 (-58.0818, -43.0013) -> (-58.5149, -43.0013)
  line L446 (-58.5149, -43.0013) -> (-58.5149, -42.6667)
  line L447 (-58.5149, -42.6667) -> (-57.6773, -42.6667)
  line L448 (-57.6773, -42.6667) -> (-57.6773, -45.1355)
  line L449 (-57.6747, -42.2674) -> (-58.1337, -42.2674)
  line L450 (-58.1337, -42.2674) -> (-58.1337, -41.8473)
  line L451 (-58.1337, -41.8473) -> (-57.6747, -41.8473)
  line L452 (-57.6747, -41.8473) -> (-57.6747, -42.2674)
  line L453 (-56.6789, -45.068) -> (-57.0835, -45.068)
  line L454 (-57.0835, -45.068) -> (-57.0835, -42.6667)
  line L455 (-57.0835, -42.6667) -> (-56.6789, -42.6667)
  line L456 (-56.6789, -42.6667) -> (-56.6789, -45.068)
  line L457 (-56.6504, -42.2674) -> (-57.1094, -42.2674)
  line L458 (-57.1094, -42.2674) -> (-57.1094, -41.8473)
  line L459 (-57.1094, -41.8473) -> (-56.6504, -41.8473)
  line L460 (-56.6504, -41.8473) -> (-56.6504, -42.2674)
  spline S529 degree 2 poles (-53.7875, -45.1251) (-54.135, -45.1251) (-54.6225, -44.9799) (-54.8378, -44.8761) knots 0 0 0 1 2 2 2
  line L461 (-54.8378, -44.8761) -> (-54.8378, -44.3419)
  line L462 (-54.8378, -44.3419) -> (-54.8066, -44.3419)
  spline S530 degree 2 poles (-54.8066, -44.3419) (-54.5966, -44.539) (-54.065, -44.7569) (-53.8186, -44.7569) knots 0 0 0 1 2 2 2
  spline S531 degree 2 poles (-53.8186, -44.7569) (-53.466, -44.7569) (-53.1055, -44.4638) (-53.1055, -44.2227) knots 0 0 0 1 2 2 2
  spline S532 degree 2 poles (-53.1055, -44.2227) (-53.1055, -44.0308) (-53.2948, -43.7922) (-53.4997, -43.7325) knots 0 0 0 1 2 2 2
  spline S533 degree 2 poles (-53.4997, -43.7325) (-53.6475, -43.6911) (-53.8938, -43.634) (-54.078, -43.5873) knots 0 0 0 1 2 2 2
  spline S534 degree 2 poles (-54.078, -43.5873) (-54.2439, -43.5432) (-54.5058, -43.411) (-54.607, -43.3047) knots 0 0 0 1 2 2 2
  spline S535 degree 2 poles (-54.607, -43.3047) (-54.7055, -43.1984) (-54.8144, -42.9131) (-54.8144, -42.7264) knots 0 0 0 1 2 2 2
  spline S536 degree 2 poles (-54.8144, -42.7264) (-54.8144, -42.3374) (-54.2076, -41.811) (-53.7383, -41.811) knots 0 0 0 1 2 2 2
  spline S537 degree 2 poles (-53.7383, -41.811) (-53.4686, -41.811) (-52.9914, -41.9173) (-52.7865, -42.0184) knots 0 0 0 1 2 2 2
  line L463 (-52.7865, -42.0184) -> (-52.7865, -42.5267)
  line L464 (-52.7865, -42.5267) -> (-52.8177, -42.5267)
  spline S538 degree 2 poles (-52.8177, -42.5267) (-52.9707, -42.3867) (-53.4478, -42.1792) (-53.7097, -42.1792) knots 0 0 0 1 2 2 2
  spline S539 degree 2 poles (-53.7097, -42.1792) (-54.0053, -42.1792) (-54.371, -42.4567) (-54.371, -42.6823) knots 0 0 0 1 2 2 2
  spline S540 degree 2 poles (-54.371, -42.6823) (-54.371, -42.8846) (-54.1558, -43.1257) (-53.9535, -43.1802) knots 0 0 0 1 2 2 2
  spline S541 degree 2 poles (-53.9535, -43.1802) (-53.8186, -43.2165) (-53.4271, -43.3099) (-53.2974, -43.3488) knots 0 0 0 1 2 2 2
  spline S542 degree 2 poles (-53.2974, -43.3488) (-52.9681, -43.4499) (-52.6621, -43.857) (-52.6621, -44.1552) knots 0 0 0 1 2 2 2
  spline S543 degree 2 poles (-52.6621, -44.1552) (-52.6621, -44.3445) (-52.8151, -44.7076) (-52.9525, -44.8347) knots 0 0 0 1 2 2 2
  spline S544 degree 2 poles (-52.9525, -44.8347) (-53.1055, -44.9747) (-53.4945, -45.1251) (-53.7875, -45.1251) knots 0 0 0 1 2 2 2
  spline S545 degree 2 poles (-50.922, -44.8139) (-50.9713, -44.8502) (-51.1373, -44.9799) (-51.2151, -45.0188) knots 0 0 0 1 2 2 2
  spline S546 degree 2 poles (-51.2151, -45.0188) (-51.3214, -45.0758) (-51.5211, -45.1355) (-51.7026, -45.1355) knots 0 0 0 1 2 2 2
  spline S547 degree 2 poles (-51.7026, -45.1355) (-51.8504, -45.1355) (-52.1175, -45.024) (-52.2186, -44.9228) knots 0 0 0 1 2 2 2
  spline S548 degree 2 poles (-52.2186, -44.9228) (-52.3146, -44.8243) (-52.4313, -44.5338) (-52.4313, -44.3731) knots 0 0 0 1 2 2 2
  spline S549 degree 2 poles (-52.4313, -44.3731) (-52.4313, -44.1241) (-52.2212, -43.7714) (-51.993, -43.6703) knots 0 0 0 1 2 2 2